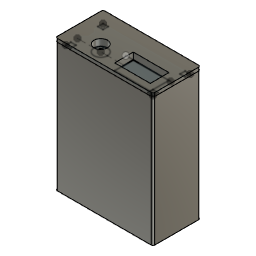
pcb holder v5 (Autodesk Fusion 360 design; units mm, degrees)
Autodesk Fusion 360 part; units mm, degrees
sketch "Sketch1" plane through (0, 0, 0) normal (0, 0, 1) x (1, 0, 0)
  line L0 (0, 0) -> (51.5, 0)
  line L1 (51.5, 0) -> (51.5, -22)
  line L2 (51.5, -22) -> (0, -22)
  line L3 (0, -22) -> (0, 0)
  line L4 (0, -8) -> (2, -8)
  line L5 (0, -9.6) -> (2, -9.6)
  line L6 (51.5, -9.6) -> (49.5, -9.6)
  line L7 (51.5, -8) -> (49.5, -8)
  line L8 (2, -9.6) -> (2, -10.6)
  line L9 (2, -10.6) -> (0, -12.6)
  line L10 (2, -10.6) -> (4.8284, -10.6) construction
  line L11 (2, -8) -> (2, -7)
  line L12 (2, -7) -> (0, -5)
  line L13 (2, -7) -> (4.8284, -7) construction
  line L14 (49.5, -8) -> (49.5, -7)
  line L15 (49.5, -9.6) -> (49.5, -10.6)
  line L16 (49.5, -10.6) -> (51.5, -12.6)
  line L17 (49.5, -10.6) -> (51.8284, -10.6) construction
  line L18 (49.5, -7) -> (51.5, -5)
  line L19 (49.5, -7) -> (51.8284, -7) construction
  line L20 (-3, -25) -> (-3, 3)
  line L21 (-3, 3) -> (54.5, 3)
  line L22 (54.5, 3) -> (54.5, -25)
  line L23 (54.5, -25) -> (-3, -25)
  point P0 (0, -11)
  point P1 (51.5, -11)
  dimension "d1" = 22
  dimension "d2" = 51.5
  dimension "d3" = 2
  dimension "d4" = 2
  dimension "d5" = 2
  dimension "d7" = 2
  dimension "d10" = 3
  dimension "d12" = 1
  dimension "d13" = 135
  dimension "d14" = 1
  dimension "d15" = 135
  dimension "d16" = 1
  dimension "d17" = 1
  dimension "d18" = 45
  dimension "d19" = 45
  dimension "d20" = -3
  dimension "d23" = 3
  dimension "d26" = 1.6
  dimension "d27" = 1.6
  constraint horizontal L0
  constraint vertical L1
  constraint horizontal L2
  constraint vertical L3
  constraint coincident L0.start L3.end
  constraint midpoint L3 P0
  constraint midpoint L1 P1
  constraint coincident L3 L4.start
  constraint perpendicular L3 L4
  constraint coincident L3 L5.start
  constraint perpendicular L3 L5
  constraint coincident L1 L6.start
  constraint perpendicular L1 L6
  constraint coincident L1 L7.start
  constraint perpendicular L1 L7
  constraint perpendicular L5 L8
  constraint horizontal L10
  constraint coincident L3 L9.end
  constraint perpendicular L4 L11
  constraint horizontal L13
  constraint coincident L3 L12.end
  constraint perpendicular L7 L14
  constraint perpendicular L6 L15
  constraint horizontal L17
  constraint coincident L1 L16.end
  constraint horizontal L19
  constraint coincident L1 L18.end
  measures "d1" distance of L0.start L2.end
  measures "d2" distance of L0.start L0.end
  measures "d3" distance of L5.start L5.end
  measures "d4" distance of L4.start L4.end
  measures "d5" distance of L7.start L7.end
  measures "d7" distance of L6.start L6.end
  measures "d10" distance of P0 L4
  measures "d12" distance of L5.end L8.end
  measures "d13" angle of L9 L10
  measures "d14" distance of L4.end L11.end
  measures "d15" angle of L12 L13
  measures "d16" distance of L7.end L14.end
  measures "d17" distance of L6.end L15.end
  measures "d18" angle of L16 L17
  measures "d19" angle of L18 L19
  measures "d23" distance of P1 L7
  measures "d26" distance of L4 L5
  measures "d27" distance of L6 L7
extrude "Extrude1" add sketch "Sketch1" along normal blind 73 contours L3 L4 L11 L12 | L1 L7 L14 L18 | L3 L5 L8 L9 | L1 L6 L15 L16 | L20 L21 L22 L23 makes body 1
fillet "Fillet1" radius 1 4 edges at (-3, -25, 36.5) (54.5, -25, 36.5) (54.5, 3, 36.5) (-3, 3, 36.5) on bodies 1
sketch "Sketch2" plane through (0, 0, 0) normal (0, 0, -1) x (1, 0, 0)
  line L0 (51.5, 8) -> (49.5, 8)
  line L1 (49.5, 8) -> (49.5, 7)
  line L2 (49.5, 7) -> (51.5, 5)
  line L3 (51.5, 5) -> (51.5, 0)
  line L4 (51.5, 0) -> (0, 0)
  line L5 (0, 0) -> (0, 5)
  line L6 (0, 5) -> (2, 7)
  line L7 (2, 7) -> (2, 8)
  line L8 (2, 8) -> (0, 8)
  line L9 (0, 8) -> (0, 9.6)
  line L10 (0, 9.6) -> (2, 9.6)
  line L11 (2, 9.6) -> (2, 10.6)
  line L12 (2, 10.6) -> (0, 12.6)
  line L13 (51.5, 22) -> (51.5, 12.6)
  line L14 (51.5, 12.6) -> (49.5, 10.6)
  line L15 (49.5, 10.6) -> (49.5, 9.6)
  line L16 (49.5, 9.6) -> (51.5, 9.6)
  line L17 (51.5, 9.6) -> (51.5, 8)
  arc A0 (-3, -2) -> (-2, -3) centre (-2, -2) ccw
  line L18 (-2, -3) -> (53.5, -3)
  arc A1 (53.5, -3) -> (54.5, -2) centre (53.5, -2) ccw
  line L19 (54.5, -2) -> (54.5, 24)
  arc A2 (54.5, 24) -> (53.5, 25) centre (53.5, 24) ccw
  line L20 (53.5, 25) -> (-2, 25)
  arc A3 (-2, 25) -> (-3, 24) centre (-2, 24) ccw
  line L21 (-3, 24) -> (-3, -2)
  arc A4 (-3, -2) -> (-2, -3) centre (-2, -2) ccw
  line L22 (-3, -2) -> (-3, 24)
  arc A5 (53.5, -3) -> (54.5, -2) centre (53.5, -2) ccw
  line L23 (54.5, 24) -> (54.5, -2)
  arc A6 (54.5, 24) -> (53.5, 25) centre (53.5, 24) ccw
  arc A7 (-2, 25) -> (-3, 24) centre (-2, 24) ccw
  line L24 (49.5, 7) -> (49.5, 8)
  line L25 (51.5, 5) -> (49.5, 7)
  line L26 (51.5, 0) -> (51.5, 5)
  line L27 (0, 0) -> (51.5, 0)
  line L28 (0, 5) -> (0, 0)
  line L29 (2, 7) -> (0, 5)
  line L30 (2, 8) -> (2, 7)
  line L31 (0, 8) -> (2, 8)
  line L32 (0, 9.6) -> (0, 8)
  line L33 (2, 9.6) -> (0, 9.6)
  line L34 (2, 10.6) -> (2, 9.6)
  line L35 (0, 12.6) -> (2, 10.6)
  line L36 (51.5, 22) -> (0, 22)
  line L37 (51.5, 12.6) -> (51.5, 22)
  line L38 (49.5, 10.6) -> (51.5, 12.6)
  line L39 (49.5, 9.6) -> (49.5, 10.6)
  line L40 (51.5, 9.6) -> (49.5, 9.6)
  line L41 (51.5, 8) -> (51.5, 9.6)
  line L42 (49.5, 8) -> (51.5, 8)
  line L43 (-2, 25) -> (53.5, 25)
  line L44 (53.5, -3) -> (-2, -3)
extrude "Extrude2" add sketch "Sketch2" along normal blind 3 bodies 1
extrude "Extrude3" add 1 faces at (35, -6.3333, -3) along direction (0, 0, 1) blind 2 from surface at 76 separate body on bodies 1 makes body 2
extrude "Extrude4" add 1 faces at (35, -6.3333, 73) along direction (0, 0, -1) blind 2 on bodies 2 bodies 2
combine "Combine1" operation cut target body 2 tool bodies 1 keep tools
move_face "OffsetFaces1" offset -2 1 faces at (0, -9.0667, 71.6667) on bodies 2
move_face "OffsetFaces2" offset -2 1 faces at (51.5, -8.5333, 71.6667) on bodies 2
sketch "Sketch3" plane through (0, 0, 71) normal (0, 0, -1) x (1, 0, 0)
  line L0 (49.5, 7) -> (49.5, 10.6)
  line L1 (49.5, 10.6) -> (51.5, 12.6)
  line L2 (51.5, 12.6) -> (51.5, 22)
  line L3 (51.5, 22) -> (0, 22)
  line L4 (0, 22) -> (0, 12.6)
  line L5 (0, 12.6) -> (2, 10.6)
  line L6 (2, 10.6) -> (2, 7)
  line L7 (2, 7) -> (0, 5)
  line L8 (0, 5) -> (0, 0)
  line L9 (0, 0) -> (51.5, 0)
  line L10 (51.5, 0) -> (51.5, 5)
  line L11 (51.5, 5) -> (49.5, 7)
  line L12 (49.5, 9.6) -> (23.0305, 9.6)
  line L13 (48.5, 9.6) -> (48.5, 20.6)
  line L14 (27.5, 9.6) -> (27.5, 20.6)
  line L15 (27.5, 20.6) -> (48.5, 20.6)
  line L16 (27.5, 15.1) -> (0, 15.1) construction
  circle A0 centre (13.75, 15.1) radius 3.95
  line L17 (0, 22) -> (3, 22)
  line L18 (3, 22) -> (3, 19)
  line L19 (3, 19) -> (0, 19)
  line L20 (0, 19) -> (0, 22)
  line L21 (0, 0) -> (3, 0)
  line L22 (3, 0) -> (3, 3)
  line L23 (3, 3) -> (0, 3)
  line L24 (0, 3) -> (0, 0)
  line L25 (51.5, 0) -> (48.5, 0)
  line L26 (48.5, 0) -> (48.5, 3)
  line L27 (48.5, 3) -> (51.5, 3)
  line L28 (51.5, 3) -> (51.5, 0)
  line L29 (51.5, 22) -> (48.5, 22)
  line L30 (48.5, 22) -> (48.5, 19)
  line L31 (48.5, 19) -> (51.5, 19)
  line L32 (51.5, 19) -> (51.5, 22)
  dimension "d38" = 1
  dimension "d39" = 11
  dimension "d40" = 1
  dimension "d41" = 11
  dimension "d42" = 21
  dimension "d43" = 7.9
  dimension "d46" = 3
  dimension "d47" = 3
  dimension "d48" = 3
  dimension "d49" = 3
  dimension "d50" = 3
  dimension "d51" = 3
  dimension "d52" = 3
  dimension "d53" = 3
  constraint coincident L0 L12.start
  constraint perpendicular L0 L12
  constraint coincident L12 L13.start
  constraint perpendicular L12 L13
  constraint coincident L12 L14.start
  constraint perpendicular L12 L14
  constraint midpoint L14 L16.start
  constraint coincident L4 L16.end
  constraint perpendicular L4 L16
  constraint midpoint L16 A0.centre
  constraint horizontal L17
  constraint vertical L18
  constraint horizontal L19
  constraint vertical L20
  constraint coincident L3.end L4.start
  constraint horizontal L21
  constraint vertical L22
  constraint horizontal L23
  constraint vertical L24
  constraint coincident L8.end L9.start
  constraint horizontal L25
  constraint vertical L26
  constraint horizontal L27
  constraint vertical L28
  constraint coincident L9.end L10.start
  constraint horizontal L29
  constraint vertical L30
  constraint horizontal L31
  constraint vertical L32
  constraint coincident L2.end L3.start
  measures "d38" distance of L0.end L12
  measures "d39" distance of L13.start L13.end
  measures "d40" distance of L0 L13
  measures "d41" distance of L14.start L14.end
  measures "d42" distance of L13 L14
  measures "d43" diameter of A0
  measures "d46" distance of L3.end L19.end
  measures "d47" distance of L3.end L17.end
  measures "d48" distance of L8.end L23.end
  measures "d49" distance of L8.end L21.end
  measures "d50" distance of L9.end L25.end
  measures "d51" distance of L9.end L27.end
  measures "d52" distance of L2.end L29.end
  measures "d53" distance of L2.end L31.end
extrude "Extrude5" cut sketch "Sketch3" against normal blind 5 contours L12 L13 L14 L15 L30 | A0 bodies 2
extrude "Extrude6" add sketch "Sketch3" along normal blind 3 contours L9 L10 L25 L26 L27 L28 | L2 L3 L13 L29 L30 L31 L32 | L8 L9 L21 L22 L23 L24 | L3 L4 L17 L18 L19 L20 bodies 2
equation "d15 = 45 deg + 90 deg"
